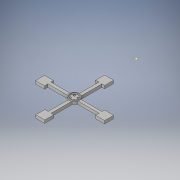
# Autodesk Inventor part: Part7
Saved by Autodesk Inventor 2016 (Build 200138000, 138)
## iProperties
Created: 2016-03-23
Part Number: Part7
Material: Generic
Document SubType Name: Modeling
Designer: Dhivya Sukumar
Density: 1 g/cm^3
Appearance: Default
Author: Dhivya Sukumar
Autodesk Inventor part; units mm, degrees
ref_plane "YZ Plane" through (0, 0, 0) normal (1, 0, 0) x (0, 1, 0)
ref_plane "XZ Plane" through (0, 0, 0) normal (0, 1, 0) x (-1, 0, 0)
ref_plane "XY Plane" through (0, 0, 0) normal (0, 0, 1) x (1, 0, 0)
sketch "Sketch1" plane through (0, 0, 0) normal (0, 1, 0) x (-1, 0, 0)
  line L0 (-9.3478, 139.075) -> (-9.3478, 139.4112)
  line L1 (2.5473, 133.0612) -> (47.8022, 133.0612)
  line L2 (47.8022, 133.0612) -> (47.8022, 139.4112)
  line L3 (47.8022, 139.4112) -> (3.1135, 139.4112)
  line L4 (-2.9978, 139.4112) -> (-2.9978, 139.075)
  line L5 (-13.4187, 133.0612) -> (-60.1478, 133.0612)
  line L6 (-60.1478, 133.0612) -> (-60.1478, 139.075)
  line L7 (-60.1478, 139.075) -> (-14.0737, 139.075)
  line L8 (-9.3478, 189.875) -> (-2.9978, 189.875)
  line L9 (-9.3478, 128.9903) -> (-9.3478, 82.2612)
  line L10 (-9.3478, 82.2612) -> (-2.9978, 82.2612)
  line L11 (-2.9978, 82.2612) -> (-2.9978, 128.4241)
  line L12 (-14.9607, 189.7858) -> (4.0893, 189.7858)
  line L13 (4.0893, 189.7858) -> (4.0893, 208.8358)
  line L14 (4.0893, 208.8358) -> (-14.9607, 208.8358)
  line L15 (-14.9607, 208.8358) -> (-14.9607, 189.7858)
  line L16 (-60.1478, 146.4982) -> (-79.1978, 146.4982)
  line L17 (-79.1978, 146.4982) -> (-79.1978, 127.4482)
  line L18 (-79.1978, 127.4482) -> (-60.1478, 127.4482)
  line L19 (-60.1478, 127.4482) -> (-60.1478, 146.4982)
  line L20 (4.0893, 82.3504) -> (-14.9607, 82.3504)
  line L21 (-14.9607, 82.3504) -> (-14.9607, 63.3004)
  line L22 (-14.9607, 63.3004) -> (4.0893, 63.3004)
  line L23 (4.0893, 63.3004) -> (4.0893, 82.3504)
  line L24 (47.8022, 146.4982) -> (66.8522, 146.4982)
  line L25 (66.8522, 146.4982) -> (66.8522, 127.4482)
  line L26 (66.8522, 127.4482) -> (47.8022, 127.4482)
  line L27 (47.8022, 127.4482) -> (47.8022, 146.4982)
  circle A0 centre (-5.4357, 136.9732) radius 8.89
  line L28 (-9.3478, 139.075) -> (-9.3478, 139.4112)
  line L29 (-9.3478, 144.9562) -> (-9.3478, 189.875)
  line L30 (-2.9978, 189.875) -> (-2.9978, 145.5224)
  line L31 (-2.9978, 139.4112) -> (-2.9978, 139.075)
  constraints: 64 end point, 16 parallel, 11 perpendicular, 4 horizontal, 1 point on line, 10 other
extrude "Extrusion1" add sketch "Sketch1" along normal blind 6.35
sketch "Sketch2" plane through (0, 6.35, 0) normal (0, 1, 0) x (1, 0, 0)
  line L0 (-47.8022, -139.4112) -> (-3.1135, -139.4112) projected
  circle A0 centre (5.4822, -136.8972) radius 8.9557
  circle A1 centre (5.4822, -136.8972) radius 10.5259
  point P0 (0, 0)
  constraints: 1 centre point, 3 other
extrude "Extrusion2" add sketch "Sketch2" along normal blind 2.794
sketch "Sketch3" plane through (0, 6.35, 0) normal (0, 1, 0) x (1, 0, 0)
  point P0 (0, 0)
hole "Hole1" at (1.0354, 0, 140.8984) direction (0, 1, 0) diameter 3.81 end through all counterbore diameter 4.826 counterbore depth 3.81
hole "Hole2" at (9.6697, 0, 132.9413) direction (0, 1, 0) diameter 3.81 end through all counterbore diameter 4.826 counterbore depth 3.81
hole "Hole3" at (9.5106, 0, 141.2132) direction (0, 1, 0) diameter 3.81 end through all counterbore diameter 4.826 counterbore depth 3.81
hole "Hole4" at (1.3978, 0, 132.6231) direction (0, 1, 0) diameter 3.81 end through all counterbore diameter 4.826 counterbore depth 3.81
body "Solid1"
